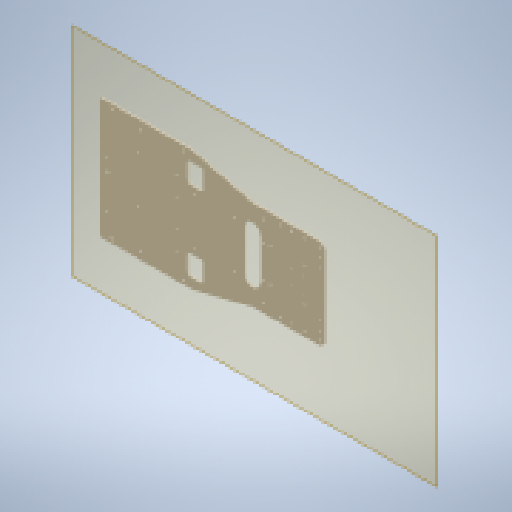
# Autodesk Inventor part: Base2
Saved by Autodesk Inventor 2023 (Build 270158000, 158)
## iProperties
Created: 2023-12-03
Part Number: Base2
Material: Genérico
Document SubType Name: Modeling
Designer: ASUS
Density: 1 g/cm^3
Appearance: Valor por defecto
Author: ASUS
Autodesk Inventor part; units mm, degrees
ref_plane "YZ Plane" through (0, 0, 0) normal (1, 0, 0) x (0, 1, 0)
ref_plane "XZ Plane" through (0, 0, 0) normal (0, 1, 0) x (-1, 0, 0)
ref_plane "XY Plane" through (0, 0, 0) normal (0, 0, 1) x (1, 0, 0)
ref_plane "Plano de trabajo1" through (0, 0, 0) normal (0, 0, 1) x (1, 0, 0)
sketch "Boceto1" plane through (0, 0, 0) normal (0, 0, 1) x (1, 0, 0)
  line L0 (75, -56) -> (80, -51)
  line L1 (80, -51) -> (80, 51)
  line L2 (80, 51) -> (75, 56)
  line L3 (75, 56) -> (-10, 56)
  line L4 (-10, 56) -> (-84.9998, 75)
  line L5 (-84.9998, 75) -> (-200, 75)
  line L6 (-200, 75) -> (-200, -75)
  line L7 (-200, -75) -> (-85, -75)
  line L8 (-85, -75) -> (-10.0003, -56)
  line L9 (-10.0003, -56) -> (75, -56)
  circle A0 centre (-184.9999, -70) radius 1.5
  circle A1 centre (25, -50) radius 1.5
  circle A2 centre (25, 50) radius 1.5
  line L10 (-91, 40) -> (-91, 59)
  arc A3 (-88, 62) -> (-91, 59) centre (-88, 59) ccw
  line L11 (-88, 62) -> (-74, 62)
  arc A4 (-71, 59) -> (-74, 62) centre (-74, 59) ccw
  line L12 (-71, 59) -> (-71, 40)
  arc A5 (-74, 37) -> (-71, 40) centre (-74, 40) ccw
  line L13 (-74, 37) -> (-88, 37)
  arc A6 (-91, 40) -> (-88, 37) centre (-88, 40) ccw
  line L14 (-91, -59) -> (-91, -40)
  arc A7 (-88, -37) -> (-91, -40) centre (-88, -40) ccw
  line L15 (-88, -37) -> (-74, -37)
  arc A8 (-71, -40) -> (-74, -37) centre (-74, -40) ccw
  line L16 (-71, -40) -> (-71, -59)
  arc A9 (-74, -62) -> (-71, -59) centre (-74, -59) ccw
  line L17 (-74, -62) -> (-88, -62)
  arc A10 (-91, -59) -> (-88, -62) centre (-88, -59) ccw
  line L18 (-20, -25) -> (-20, 25)
  line L19 (0, 25) -> (0, -25)
  circle A11 centre (-10, 25) radius 10
  circle A12 centre (-10, -25) radius 10
  circle A13 centre (-147.9, 65) radius 1.5
  circle A14 centre (-153, 39) radius 1.25
  circle A15 centre (-190, 15) radius 1.25
  circle A16 centre (-189.9, 0) radius 1.5
  circle A17 centre (-190, -43) radius 1.25
  circle A18 centre (-153, -19) radius 1.25
  circle A19 centre (-147.8999, -65) radius 1.5001
  circle A20 centre (-104, -43) radius 1.25
  circle A21 centre (-81.6553, -29) radius 1.25
  circle A22 centre (-104, -19) radius 1.25
  circle A23 centre (-32.6553, -29) radius 1.25
  circle A24 centre (-104, 15) radius 1.25
  circle A25 centre (-81.6553, 29) radius 1.25
  circle A26 centre (-104, 39) radius 1.25
  circle A27 centre (-32.6553, 29) radius 1.25
  circle A28 centre (4.1, -45) radius 1.5
  circle A29 centre (4, -20) radius 1.25
  circle A30 centre (12.6404, -20.8597) radius 1.5
  circle A31 centre (4, 20) radius 1.25
  circle A32 centre (12.6404, 20.8597) radius 1.5
  circle A33 centre (4.1, 45) radius 1.5
  circle A34 centre (54.6, -49.9999) radius 1.5001
  circle A35 centre (75, -50) radius 1.25
  circle A36 centre (75, -40) radius 1.25
  circle A37 centre (74, -28) radius 1.25
  circle A38 centre (54.3596, -20.8597) radius 1.5
  circle A39 centre (54.1, -9.25) radius 0.75
  circle A40 centre (40.1, -9.25) radius 0.75
  circle A41 centre (39.6, 50) radius 1.5
  circle A42 centre (54.6, 50) radius 1.5
  circle A43 centre (54.3597, 20.8596) radius 1.5
  circle A44 centre (54.1, 9.25) radius 0.75
  circle A45 centre (40.1, 9.25) radius 0.75
  circle A46 centre (74, 28) radius 1.25
  circle A47 centre (75, 50) radius 1.25
  circle A48 centre (75, 40) radius 1.25
  circle A49 centre (39.6, -50) radius 1.25
  circle A50 centre (25, -50) radius 1.5
  circle A51 centre (-95, -70) radius 1.5
  circle A52 centre (-185, -70) radius 1.5
  circle A53 centre (-185, 70) radius 1.5
  circle A54 centre (-95, 70) radius 1.5
  circle A55 centre (25, 50) radius 1.5
  point P0 (26.4595, -50.3464)
  point P1 (23.6185, -50.5842)
  point P2 (0, -24.9924)
  point P3 (-20, -24.9924)
  constraints: 55 centre point, 40 end point, 16 point on circle, 2 other
extrude "Extrusión1" add sketch "Boceto1" against normal blind 2
ref_plane "Plano de trabajo2" through (-200, -75, -2.1) normal (-1, 0, 0) x (0, -1, 0)
sketch "Boceto2" plane through (-200, -75, -2.1) normal (-1, 0, 0) x (0, -1, 0)
  line L0 (-150, -12.9) -> (-150, 0.1)
  line L1 (-145, -17.9) -> (-5, -17.9)
  line L2 (-125, -8.4) -> (-25, -8.4)
  line L3 (-25, -15.4) -> (-125, -15.4)
  line L4 (-125, -15.4) -> (-125, -8.4)
  circle A0 centre (-130, -11.9) radius 1.5
  line L5 (-25, -8.4) -> (-25, -15.4)
  circle A1 centre (-20, -11.9) radius 1.5
  line L6 (0, -12.9) -> (0, 0.1)
  line L7 (0, 0.1) -> (-150, 0.1)
  arc A2 (-150, -12.9) -> (-145, -17.9) centre (-145, -12.9) ccw
  arc A3 (-5, -17.9) -> (0, -12.9) centre (-5, -12.9) ccw
  point P0 (-75, 2.1)
  dimension "d2" = 5
  constraints: 16 end point, 4 centre point, 4 point on circle, 4 tangent, 1 equal radius
  measures "d2" radius of A2
extrude "Extrusión2" add sketch "Boceto2" against normal blind 2
fillet "Empalme1" radius 2 1 edges at (-200, 0, 0)
